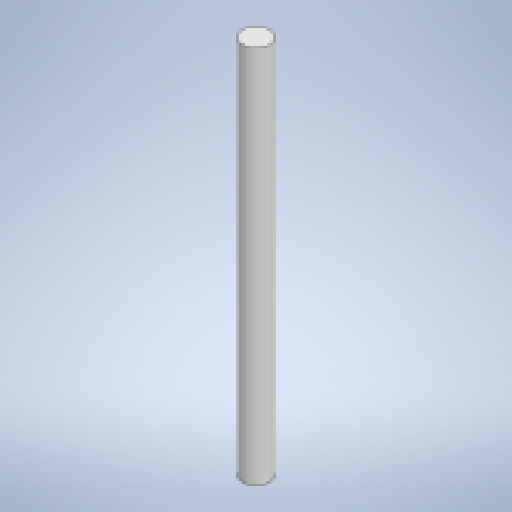
# Autodesk Inventor part: Вал ведущей шестерни
Saved by Autodesk Inventor 2025 (Build 290162010, 162A)
## iProperties
Created: 2025-08-20
Part Number: Вал ведущей шестерни
Material: Generic
Document SubType Name: Modeling
Designer: pokla
Density: 1 g/cm^3
Appearance: Default
Author: pokla
Autodesk Inventor part; units mm, degrees
ref_plane "YZ Plane" through (0, 0, 0) normal (1, 0, 0) x (0, 1, 0)
ref_plane "XZ Plane" through (0, 0, 0) normal (0, 1, 0) x (-1, 0, 0)
ref_plane "XY Plane" through (0, 0, 0) normal (0, 0, 1) x (1, 0, 0)
sketch "Sketch1" plane through (0, 0, 0) normal (0, 1, 0) x (-1, 0, 0)
  line L0 (0, 0) -> (0, 576.4967)
  line L1 (0, 0) -> (-17.5, 0)
  line L2 (-17.5, 0) -> (-17.5, 500)
  line L3 (-17.5, 500) -> (0, 500)
  line L4 (0, 500) -> (0, 0)
  point P0 (0, 500)
  dimension "d2" = 500
  dimension "d4" = 35
  constraints: 10 end point, 2 parallel, 1 horizontal, 1 perpendicular, 1 point on line, 1 vertical
  measures "d2" distance of L1.end L2.end
  measures "d4" diameter of L2 L0
revolve "Revolution1" add sketch "Sketch1" angle 360 about axis through (0, 0, 0) along (0, 0, 1)
body "Solid1"
